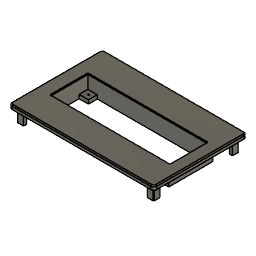
Aero Brick - Top (Autodesk Fusion 360 design; units mm, degrees)
Autodesk Fusion 360 part; units mm, degrees
sketch "Sketch1" plane through (0, 0, 0) normal (0, 0, 1) x (1, 0, 0)
  line L0 (0, 0) -> (107, 0)
  line L1 (107, 0) -> (107, 67)
  line L2 (107, 67) -> (0, 67)
  line L3 (0, 67) -> (0, 0)
  line L4 (-3, 67) -> (-3, 70)
  line L5 (-3, 70) -> (0, 70)
  line L6 (110, 0) -> (110, -3)
  line L7 (110, -3) -> (107, -3)
  line L8 (-3, 70) -> (110, 70)
  line L9 (110, 70) -> (110, -3)
  line L10 (110, -3) -> (-3, -3)
  line L11 (-3, -3) -> (-3, 70)
  dimension "d1" = 67
  dimension "d2" = 107
  dimension "d3" = 3
  dimension "d4" = 3
  dimension "d5" = 3
  constraint horizontal L0
  constraint vertical L1
  constraint horizontal L2
  constraint vertical L3
  constraint coincident L0.start L3.end
  constraint vertical L4
  constraint horizontal L5
  constraint vertical L6
  constraint horizontal L7
  constraint horizontal L8
  constraint vertical L9
  constraint horizontal L10
  constraint vertical L11
  measures "d1" distance of L0.start L2.end
  measures "d2" distance of L0.start L0.end
  measures "d3" distance of L2.end L4.start
  measures "d4" distance of L0.end L6.start
  measures "d5" distance of L0.end L7.end
extrude "Extrude1" add sketch "Sketch1" along normal blind 3
extrude "Extrude2" add sketch "Sketch1" along normal blind 3 contours L0 L1 L2 L3
fillet "Fillet1" radius 2.5 4 edges at (-3, 70, 1.5) (110, 70, 1.5) (110, -3, 1.5) (-3, -3, 1.5)
sketch "Sketch2" plane through (0, 0, 0) normal (0, 0, 1) x (1, 0, 0)
  line L0 (117.8476, 33.4729) -> (-7.2698, 33.4729)
  line L1 (53.5, 5) -> (53.5, 52.788)
  line L2 (0, 67) -> (0, 0)
  line L3 (2.75, 2.75) -> (2.75, 5.25)
  line L4 (2.75, 5.25) -> (0.25, 5.25)
  line L5 (0.25, 5.25) -> (0.25, 0.25)
  line L6 (0, 0) -> (107, 0)
  line L7 (0.25, 0.25) -> (5.25, 0.25)
  line L8 (5.25, 0.25) -> (5.25, 2.75)
  line L9 (5.25, 2.75) -> (2.75, 2.75)
  line L10 (5.25, 66.6957) -> (5.25, 64.1957)
  line L11 (5.25, 64.1957) -> (2.75, 64.1957)
  line L12 (2.75, 64.1957) -> (2.75, 61.6957)
  line L13 (2.75, 61.6957) -> (0.25, 61.6957)
  line L14 (0.25, 61.6957) -> (0.25, 66.6957)
  line L15 (0.25, 66.6957) -> (5.25, 66.6957)
  line L16 (101.75, 0.25) -> (101.75, 2.75)
  line L17 (106.75, 0.25) -> (101.75, 0.25)
  line L18 (106.75, 5.25) -> (106.75, 0.25)
  line L19 (104.25, 5.25) -> (106.75, 5.25)
  line L20 (104.25, 2.75) -> (104.25, 5.25)
  line L21 (101.75, 2.75) -> (104.25, 2.75)
  line L22 (101.75, 64.1957) -> (104.25, 64.1957)
  line L23 (101.75, 66.6957) -> (101.75, 64.1957)
  line L24 (106.75, 66.6957) -> (101.75, 66.6957)
  line L25 (106.75, 61.6957) -> (106.75, 66.6957)
  line L26 (104.25, 61.6957) -> (106.75, 61.6957)
  line L27 (104.25, 64.1957) -> (104.25, 61.6957)
  line L28 (0.25, 5.25) -> (10.25, 5.25)
  line L29 (10.25, 5.25) -> (10.25, 12.25)
  line L30 (10.25, 12.25) -> (0.25, 12.25)
  line L31 (0.25, 12.25) -> (0.25, 5.25)
  line L32 (0.25, 61.6957) -> (10.25, 61.6957)
  line L33 (10.25, 61.6957) -> (10.25, 54.6957)
  line L34 (10.25, 54.6957) -> (0.25, 54.6957)
  line L35 (0.25, 54.6957) -> (0.25, 61.6957)
  dimension "d14" = 53.5
  dimension "d16" = 5
  dimension "d17" = 0.25
  dimension "d19" = 5
  dimension "d55" = 10
  dimension "d56" = 7
  dimension "d57" = 10
  dimension "d58" = 7
  constraint vertical L1
  constraint vertical L3
  constraint horizontal L4
  constraint vertical L5
  constraint horizontal L7
  constraint vertical L8
  constraint horizontal L9
  constraint symmetric L0 L5.end L14.end
  constraint symmetric L0 L3.end L12.end
  constraint symmetric L0 L4.end L13.end
  constraint symmetric L0 L7.end L10.start
  constraint symmetric L0 L8.end L10.end
  constraint symmetric L0 L3.start L11.end
  constraint symmetric L1 L5.end L17.start
  constraint symmetric L1 L3.end L19.start
  constraint symmetric L1 L4.end L18.start
  constraint symmetric L1 L7.end L16.start
  constraint symmetric L1 L8.end L16.end
  constraint symmetric L1 L3.start L20.start
  constraint symmetric L1 L10.start L23.start
  constraint symmetric L1 L10.end L22.start
  constraint symmetric L1 L11.end L22.end
  constraint symmetric L1 L12.end L26.start
  constraint symmetric L1 L13.end L25.start
  constraint symmetric L1 L14.end L24.start
  constraint horizontal L28
  constraint vertical L29
  constraint horizontal L30
  constraint vertical L31
  constraint horizontal L32
  constraint vertical L33
  constraint horizontal L34
  constraint vertical L35
  measures "d14" distance of L1 L2
  measures "d16" distance of L5.end L4.end
  measures "d17" distance of L2 L5
  measures "d19" distance of L5.end L7.end
  measures "d55" distance of L4.end L28.end
  measures "d56" distance of L4.end L30.end
  measures "d57" distance of L13.end L32.end
  measures "d58" distance of L13.end L34.end
extrude "Extrude3" add sketch "Sketch2" against normal blind 10 contours L3 L4 L5 L7 L8 L9 L28 | L10 L11 L12 L13 L14 L15 L32 | L16 L17 L18 L19 L20 L21 | L22 L23 L24 L25 L26 L27
fillet "Fillet2" radius 0.5 4 edges at (106.75, 0.25, -5) (106.75, 66.6957, -5) (0.25, 66.6957, -5) (0.25, 0.25, -5)
sketch "Sketch3" plane through (0, 0, 0) normal (0, 0, -1) x (1, 0, 0)
  line L0 (101.75, -0.25) -> (106.25, -0.25)
  arc A0 (106.75, -0.75) -> (106.25, -0.25) centre (106.25, -0.75) ccw
  line L1 (106.75, -0.75) -> (106.75, -5.25)
  line L2 (106.75, -5.25) -> (104.25, -5.25)
  line L3 (104.25, -5.25) -> (104.25, -2.75)
  line L4 (104.25, -2.75) -> (101.75, -2.75)
  line L5 (101.75, -2.75) -> (101.75, -0.25)
  line L6 (2.75, -2.75) -> (2.75, -5.25)
  line L7 (2.75, -5.25) -> (0.25, -5.25)
  line L8 (0.25, -5.25) -> (0.25, -0.75)
  arc A1 (0.75, -0.25) -> (0.25, -0.75) centre (0.75, -0.75) ccw
  line L9 (0.75, -0.25) -> (5.25, -0.25)
  line L10 (5.25, -0.25) -> (5.25, -2.75)
  line L11 (5.25, -2.75) -> (2.75, -2.75)
  line L12 (104.25, -61.6957) -> (106.75, -61.6957)
  line L13 (106.75, -61.6957) -> (106.75, -66.1957)
  arc A2 (106.25, -66.6957) -> (106.75, -66.1957) centre (106.25, -66.1957) ccw
  line L14 (106.25, -66.6957) -> (101.75, -66.6957)
  line L15 (101.75, -66.6957) -> (101.75, -64.1957)
  line L16 (101.75, -64.1957) -> (104.25, -64.1957)
  line L17 (104.25, -64.1957) -> (104.25, -61.6957)
  line L18 (0.25, -61.6957) -> (2.75, -61.6957)
  line L19 (2.75, -61.6957) -> (2.75, -64.1957)
  line L20 (2.75, -64.1957) -> (5.25, -64.1957)
  line L21 (5.25, -64.1957) -> (5.25, -66.6957)
  line L22 (5.25, -66.6957) -> (0.75, -66.6957)
  arc A3 (0.25, -66.1957) -> (0.75, -66.6957) centre (0.75, -66.1957) ccw
  line L23 (0.25, -66.1957) -> (0.25, -61.6957)
  arc A4 (-0.5, 3) -> (-3, 0.5) centre (-0.5, 0.5) ccw
  line L24 (-3, 0.5) -> (-3, -67.5)
  arc A5 (-3, -67.5) -> (-0.5, -70) centre (-0.5, -67.5) ccw
  line L25 (-0.5, -70) -> (107.5, -70)
  arc A6 (107.5, -70) -> (110, -67.5) centre (107.5, -67.5) ccw
  line L26 (110, -67.5) -> (110, 0.5)
  arc A7 (110, 0.5) -> (107.5, 3) centre (107.5, 0.5) ccw
  line L27 (107.5, 3) -> (-0.5, 3)
  line L28 (8, -19.25) -> (100.5, -19.25)
  line L29 (100.5, -19.25) -> (100.5, -47.75)
  line L30 (100.5, -47.75) -> (8, -47.75)
  line L31 (8, -47.75) -> (8, -19.25)
  line L32 (54.25, -19.25) -> (54.25, 3)
  line L33 (54.25, -47.75) -> (54.25, -70)
  line L34 (102.5, -47.75) -> (102.5, -50.75)
  line L35 (102.5, -50.75) -> (100.5, -50.75)
  line L36 (5, -19.5) -> (5, -16.25)
  line L37 (5, -16.25) -> (8, -16.25)
  line L38 (5, -16.25) -> (102.5, -16.25)
  line L39 (102.5, -16.25) -> (102.5, -50.75)
  line L40 (102.5, -50.75) -> (5, -50.75)
  line L41 (5, -50.75) -> (5, -16.25)
  dimension "d25" = 28.5
  dimension "d26" = 92.5
  dimension "d27" = 7.75
  dimension "d28" = 2
  dimension "d29" = 3
  dimension "d30" = 3
  constraint horizontal L28
  constraint vertical L29
  constraint horizontal L30
  constraint vertical L31
  constraint vertical L32
  constraint midpoint L28 L32.start
  constraint coincident L27 L32.end
  constraint vertical L33
  constraint midpoint L30 L33.start
  constraint coincident L25 L33.end
  constraint equal L32 L33
  constraint vertical L34
  constraint horizontal L35
  constraint vertical L36
  constraint horizontal L37
  constraint horizontal L38
  constraint vertical L39
  constraint horizontal L40
  constraint vertical L41
  measures "d25" distance of L28.start L30.end
  measures "d26" distance of L28.start L28.end
  measures "d27" distance of L8 L31
  measures "d28" distance of L29.end L34.start
  measures "d29" distance of L29.end L35.end
  measures "d30" distance of L28.start L37.end
extrude "Extrude4" cut sketch "Sketch3" against normal blind 5 contours L28 L29 L30 L31
extrude "Extrude5" add sketch "Sketch3" along normal blind 10.5 contours L28 L29 L30 L32 L33 L34 L35 L38 L39 L40 | L28 L30 L31 L32 L33 L36 L37 L38 L40 L41
sketch "Sketch4" plane through (0, 0, -10.5) normal (0, 0, -1) x (1, 0, 0)
  line L0 (100.5, -47.75) -> (8, -47.75)
  line L1 (8, -47.75) -> (8, -19.25)
  line L2 (8, -19.25) -> (100.5, -19.25)
  line L3 (100.5, -19.25) -> (100.5, -47.75)
  line L4 (5, -50.75) -> (102.5, -50.75)
  line L5 (102.5, -50.75) -> (102.5, -16.25)
  line L6 (102.5, -16.25) -> (5, -16.25)
  line L7 (5, -16.25) -> (5, -50.75)
  circle A0 centre (11.835, -22.64) radius 0.575
  circle A1 centre (96.665, -22.64) radius 0.575
  circle A2 centre (96.665, -44.36) radius 0.575
  circle A3 centre (11.835, -44.36) radius 0.575
  line L8 (12.41, -22.64) -> (15.335, -22.64)
  line L9 (15.335, -22.64) -> (15.335, -26.14)
  line L10 (15.335, -26.14) -> (11.835, -26.14)
  line L11 (11.835, -26.14) -> (11.835, -23.215)
  line L12 (12.41, -44.36) -> (15.335, -44.36)
  line L13 (15.335, -44.36) -> (15.335, -40.86)
  line L14 (15.335, -40.86) -> (11.835, -40.86)
  line L15 (11.835, -40.86) -> (11.835, -43.785)
  line L16 (96.09, -44.36) -> (93.165, -44.36)
  line L17 (93.165, -44.36) -> (93.165, -40.86)
  line L18 (93.165, -40.86) -> (96.665, -40.86)
  line L19 (96.665, -40.86) -> (96.665, -43.785)
  line L20 (96.09, -22.64) -> (93.165, -22.64)
  line L21 (93.165, -22.64) -> (93.165, -26.14)
  line L22 (93.165, -26.14) -> (96.665, -26.14)
  line L23 (96.665, -26.14) -> (96.665, -23.215)
  line L24 (93.165, -26.14) -> (100.5, -26.14)
  line L25 (100.5, -26.14) -> (100.5, -19.25)
  line L26 (100.5, -19.25) -> (93.165, -19.25)
  line L27 (93.165, -19.25) -> (93.165, -26.14)
  line L28 (93.165, -40.86) -> (100.5, -40.86)
  line L29 (100.5, -40.86) -> (100.5, -47.75)
  line L30 (100.5, -47.75) -> (93.165, -47.75)
  line L31 (93.165, -47.75) -> (93.165, -40.86)
  line L32 (15.335, -40.86) -> (8, -40.86)
  line L33 (8, -40.86) -> (8, -47.75)
  line L34 (8, -47.75) -> (15.335, -47.75)
  line L35 (15.335, -47.75) -> (15.335, -40.86)
  line L36 (15.335, -26.14) -> (8, -26.14)
  line L37 (8, -26.14) -> (8, -19.25)
  line L38 (8, -19.25) -> (15.335, -19.25)
  line L39 (15.335, -19.25) -> (15.335, -26.14)
  dimension "d36" = 84.83
  dimension "d39" = 1.15
  dimension "d40" = 1.15
  dimension "d41" = 1.15
  dimension "d42" = 1.15
  dimension "d43" = 3.5
  dimension "d44" = 3.5
  dimension "d45" = 3.5
  dimension "d46" = 3.5
  dimension "d47" = 3.5
  dimension "d48" = 3.5
  dimension "d49" = 3.5
  dimension "d50" = 3.5
  constraint horizontal L8
  constraint vertical L9
  constraint horizontal L10
  constraint vertical L11
  constraint horizontal L12
  constraint vertical L13
  constraint horizontal L14
  constraint vertical L15
  constraint horizontal L16
  constraint vertical L17
  constraint horizontal L18
  constraint vertical L19
  constraint horizontal L20
  constraint vertical L21
  constraint horizontal L22
  constraint vertical L23
  constraint horizontal L24
  constraint vertical L25
  constraint horizontal L26
  constraint vertical L27
  constraint coincident L2.end L3.start
  constraint horizontal L28
  constraint vertical L29
  constraint horizontal L30
  constraint vertical L31
  constraint coincident L0.start L3.end
  constraint horizontal L32
  constraint vertical L33
  constraint horizontal L34
  constraint vertical L35
  constraint coincident L0.end L1.start
  constraint horizontal L36
  constraint vertical L37
  constraint horizontal L38
  constraint vertical L39
  constraint coincident L1.end L2.start
  constraint coincident A0 L11.end
  constraint coincident A0 L8.start
  constraint coincident A1 L23.end
  constraint coincident A1 L20.start
  constraint coincident A2 L19.end
  constraint coincident A2 L16.start
  constraint coincident A3 L15.end
  constraint coincident A3 L12.start
  measures "d36" distance of A0.centre A1.centre
  measures "d39" diameter of A0
  measures "d40" diameter of A1
  measures "d41" diameter of A2
  measures "d42" diameter of A3
  measures "d43" distance of A0.centre L8.end
  measures "d44" distance of A0.centre L10.end
  measures "d45" distance of A3.centre L12.end
  measures "d46" distance of A3.centre L14.end
  measures "d47" distance of A2.centre L16.end
  measures "d48" distance of A2.centre L18.end
  measures "d49" distance of A1.centre L20.end
  measures "d50" distance of A1.centre L22.end
extrude "Extrude6" add sketch "Sketch4" against normal blind 3 contours L0 L3 A2 L16 L19 L28 L29 L30 L31 | L0 L1 A3 L12 L15 L32 L33 L34 L35 | A2 L16 L17 L18 L19 L28 L31 | L2 L3 A1 L20 L23 L24 L25 L26 L27 | A3 L12 L13 L14 L15 L32 L35 | A1 L20 L21 L22 L23 L24 L27 | L1 L2 A0 L8 L11 L36 L37 L38 L39 | A0 L8 L9 L10 L11 L36 L39
fillet "Fillet3" radius 0.5 4 edges at (54.25, 19.25, 3) (54.25, 47.75, 3) (8, 33.5, 3) (100.5, 33.5, 3)
extrude "Extrude7" add sketch "Sketch2" against normal blind 7 contours L4 L28 L29 L30 L31 | L13 L32 L33 L34 L35
sketch "Sketch5" plane through (0.25, 0, 0) normal (-1, 0, 0) x (0, -1, 0)
  line L0 (-0.75, -10) -> (-0.75, 0)
  line L1 (-0.75, 0) -> (-12.25, 0)
  line L2 (-12.25, 0) -> (-12.25, -7)
  line L3 (-12.25, -7) -> (-5.25, -7)
  line L4 (-5.25, -7) -> (-5.25, -10)
  line L5 (-5.25, -10) -> (-0.75, -10)
  circle A0 centre (-8.625, -3.5) radius 5.0389
  circle A1 centre (-8.625, -3.5) radius 1.75
  circle A2 centre (-58.35, -3.5) radius 5.0569
  circle A3 centre (-58.35, -3.5) radius 1.75
  dimension "d61" = 3.5
  dimension "d62" = 3.5
  constraint coincident L2.end A0
  constraint concentric A0 A1
  constraint concentric A2 A3
  measures "d61" diameter of A1
  measures "d62" diameter of A3
extrude "Extrude8" cut sketch "Sketch5" against normal blind 7 contours A1 | A3
chamfer "Chamfer1" distance 0.8 angle 45 8 edges at (110, 33.5, 3) (109.2678, 69.2678, 3) (53.5, 70, 3) (-2.2678, 69.2678, 3) (-3, 33.5, 3) (-2.2678, -2.2678, 3) (53.5, -3, 3) (109.2678, -2.2678, 3)
equation "d14 = ( 107 / 2 ) * 1 mm"
